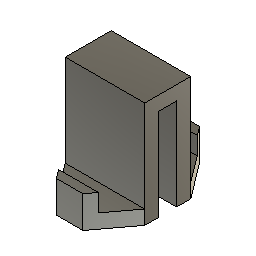
verkefni3_snagi v2 (Autodesk Fusion 360 design; units mm, degrees)
Autodesk Fusion 360 part; units mm, degrees
sketch "Sketch1" plane through (0, 0, 0) normal (0, 1, 0) x (1, 0, 0)
  line L0 (0, 0) -> (45, 0)
  line L1 (45, 0) -> (45, -60)
  line L2 (45, -60) -> (0, -60)
  line L3 (0, -60) -> (0, 0)
  dimension "d9" = 45
  dimension "d10" = 60
  constraint horizontal L0
  constraint vertical L1
  constraint horizontal L2
  constraint vertical L3
  constraint coincident L0.start L3.end
  measures "d9" distance of L1.end L2.end
  measures "d10" distance of L0.start L2.end
extrude "Extrude1" add sketch "Sketch1" against normal blind 8
sketch "Sketch3" plane through (0, 0, 0) normal (0, 1, 0) x (-1, 0, 0)
  line L0 (0, 60) -> (-45, 60)
  line L1 (-45, 60) -> (-45, 0)
  line L2 (-45, 0) -> (0, 0)
  line L3 (0, 0) -> (0, 60)
  line L4 (-45, 60) -> (0, 60)
  line L5 (0, 60) -> (0, 52)
  line L6 (0, 52) -> (-45, 52)
  line L7 (-45, 52) -> (-45, 60)
  dimension "d13" = 45
  dimension "d14" = 8
  constraint horizontal L4
  constraint vertical L5
  constraint horizontal L6
  constraint vertical L7
  constraint coincident L0.end L1.start
  measures "d13" distance of L0.end L0.start
  measures "d14" distance of L0.end L6.end
extrude "Extrude2" add sketch "Sketch3" along normal blind 18 contours L0 L1 L3 L4 L5 L6 L7
sketch "Sketch4" plane through (0, 0, 52) normal (0, 0, -1) x (1, 0, 0)
  line L0 (45, 0) -> (0, 0)
  line L1 (0, 0) -> (0, -18)
  line L2 (0, -18) -> (45, -18)
  line L3 (45, -18) -> (45, 0)
  line L4 (0, -18) -> (45, -18)
  line L5 (45, -18) -> (45, -10)
  line L6 (45, -10) -> (0, -10)
  line L7 (0, -10) -> (0, -18)
  dimension "d17" = 45
  dimension "d18" = 8
  constraint horizontal L4
  constraint vertical L5
  constraint horizontal L6
  constraint vertical L7
  constraint coincident L1.end L2.start
  measures "d17" distance of L1.end L2.end
  measures "d18" distance of L1.end L6.end
extrude "Extrude3" add sketch "Sketch4" along normal blind 52 contours L1 L2 L3 L4 L5 L6 L7
sketch "Sketch5" plane through (0, -8, 0) normal (0, -1, 0) x (1, 0, 0)
  line L0 (45, 60) -> (0, 60)
  line L1 (0, 60) -> (0, 0)
  line L2 (0, 0) -> (45, 0)
  line L3 (45, 0) -> (45, 60)
  line L4 (0, 0) -> (45, 0)
  line L5 (45, 0) -> (45, 8)
  line L6 (45, 8) -> (0, 8)
  line L7 (0, 8) -> (0, 0)
  dimension "d21" = 45
  dimension "d22" = 8
  constraint horizontal L4
  constraint vertical L5
  constraint horizontal L6
  constraint vertical L7
  constraint coincident L1.end L2.start
  measures "d21" distance of L5.end L6.end
  measures "d22" distance of L1.end L6.end
extrude "Extrude4" add sketch "Sketch5" along normal blind 20 contours L1 L2 L3 L4 L5 L6 L7
sketch "Sketch6" plane through (0, 0, 8) normal (0, 0, 1) x (-1, 0, 0)
  line L0 (-45, 8) -> (0, 8)
  line L1 (0, 8) -> (0, 28)
  line L2 (0, 28) -> (-45, 28)
  line L3 (-45, 28) -> (-45, 8)
  line L4 (-22.5, 28) -> (-30, 28)
  line L5 (-22.5, 28) -> (-15, 28)
  line L6 (-30, 28) -> (-45, 8)
  line L7 (-15, 28) -> (0, 8)
  dimension "d25" = 7.5
  dimension "d26" = 7.5
  constraint coincident L0.end L1.start
  constraint midpoint L2 L4.start
  constraint coincident L0.start L3.end
  constraint coincident L2 L4.end
  constraint parallel L2 L4
  constraint coincident L2 L5.end
  constraint parallel L2 L5
  measures "d25" distance of L4.start L4.end
  measures "d26" distance of L4.start L5.end
extrude "Extrude5" cut sketch "Sketch6" against normal blind 8 contours L2 L3 L6 | L1 L2 L7
sketch "Sketch7" plane through (0, 0, 8) normal (0, 0, 1) x (-1, 0, 0)
  line L0 (0, 8) -> (-15, 28)
  line L1 (-15, 28) -> (-30, 28)
  line L2 (-30, 28) -> (-45, 8)
  line L3 (-45, 8) -> (0, 8)
  line L4 (-15, 28) -> (-30, 28)
  line L5 (-30, 28) -> (-33.75, 23)
  line L6 (-33.75, 23) -> (-11.25, 23)
  line L7 (-11.25, 23) -> (-15, 28)
  dimension "d29" = 15
  dimension "d30" = 5
  constraint coincident L0.end L1.start
  constraint coincident L1.end L2.start
  constraint coincident L2 L5.end
  constraint parallel L2 L5
  constraint coincident L0 L6.end
  constraint horizontal L6
  measures "d29" distance of L0.end L1.end
  measures "d30" distance of L0.end L6
extrude "Extrude6" add sketch "Sketch7" along normal blind 10 contours L0 L1 L2 L4 L5 L6 L7
sketch "Sketch8" plane through (0, 18, 0) normal (0, 1, 0) x (-1, 0, 0)
  line L0 (0, 0) -> (0, 60)
  line L1 (0, 60) -> (-45, 60)
  line L2 (-45, 60) -> (-45, 0)
  line L3 (-45, 0) -> (0, 0)
  line L4 (-45, 0) -> (0, 0)
  line L5 (0, 0) -> (0, 8)
  line L6 (0, 8) -> (-45, 8)
  line L7 (-45, 8) -> (-45, 0)
  dimension "d33" = 45
  dimension "d34" = 8
  constraint horizontal L4
  constraint vertical L5
  constraint horizontal L6
  constraint vertical L7
  constraint coincident L2.end L3.start
  measures "d33" distance of L5.end L6.end
  measures "d34" distance of L2.end L6.end
extrude "Extrude7" add sketch "Sketch8" along normal blind 20 contours L0 L2 L3 L4 L5 L6 L7
sketch "Sketch9" plane through (0, 0, 8) normal (0, 0, 1) x (-1, 0, 0)
  line L0 (0, -18) -> (-45, -18)
  line L1 (-45, -18) -> (-45, -38)
  line L2 (-45, -38) -> (0, -38)
  line L3 (0, -38) -> (0, -18)
  line L4 (-22.5, -38) -> (-30, -38)
  line L5 (-22.5, -38) -> (-15, -38)
  line L6 (-15, -38) -> (0, -18)
  line L7 (-30, -38) -> (-45, -18)
  dimension "d37" = 7.5
  dimension "d38" = 7.5
  constraint midpoint L2 L4.start
  constraint coincident L0.start L3.end
  constraint coincident L0.end L1.start
  constraint coincident L2 L4.end
  constraint parallel L2 L4
  constraint coincident L2 L5.end
  measures "d37" distance of L4.start L4.end
  measures "d38" distance of L4.start L5.end
extrude "Extrude8" cut sketch "Sketch9" against normal blind 8 contours L2 L3 L6 | L1 L2 L7
sketch "Sketch10" plane through (0, 0, 8) normal (0, 0, 1) x (-1, 0, 0)
  line L0 (-15, -38) -> (0, -18)
  line L1 (0, -18) -> (-45, -18)
  line L2 (-45, -18) -> (-30, -38)
  line L3 (-30, -38) -> (-15, -38)
  line L4 (-15, -38) -> (-11.25, -33)
  line L5 (-15, -38) -> (-30, -38)
  line L6 (-30, -38) -> (-33.75, -33)
  line L7 (-11.25, -33) -> (-33.75, -33)
  dimension "d41" = 5
  constraint coincident L0.start L3.end
  constraint coincident L0 L4.end
  constraint parallel L0 L4
  constraint coincident L2 L6.end
  constraint coincident L2.end L3.start
  constraint parallel L2 L6
  constraint horizontal L7
  measures "d41" distance of L0.start L7
extrude "Extrude9" add sketch "Sketch10" along normal blind 10 contours L0 L2 L3 L4 L5 L6 L7
equation "haed = 60 mm"
equation "pinni_breidd = 15 mm"
equation "thykkt = 8 mm"
equation "haed_pinni = 10 mm"
equation "flotur = 20 mm"
equation "breidd = 3 * pinni_breidd"
equation "bil = 10 mm"
equation "pinni_lengd = 5 mm"
equation "d9 = breidd"
equation "d10 = haed"
equation "d11 = -thykkt"
equation "d13 = breidd"
equation "d14 = thykkt"
equation "d15 = bil + thykkt"
equation "d17 = breidd"
equation "d18 = thykkt"
equation "d19 = haed - thykkt"
equation "d21 = breidd"
equation "d22 = thykkt"
equation "d23 = flotur"
equation "d25 = pinni_breidd / 2"
equation "d26 = pinni_breidd / 2"
equation "d27 = -thykkt"
equation "d30 = pinni_lengd"
equation "d31 = haed_pinni"
equation "d33 = breidd"
equation "d34 = thykkt"
equation "d35 = flotur"
equation "d37 = pinni_breidd / 2"
equation "d38 = pinni_breidd / 2"
equation "d39 = -thykkt"
equation "d41 = pinni_lengd"
equation "d42 = haed_pinni"
